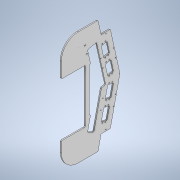
# Autodesk Inventor part: main
Saved by Autodesk Inventor 2020 (Build 240168000, 168)
## iProperties
Created: 2019-06-06
Part Number: main
Material: Generic
Document SubType Name: Modeling
Designer: Vivek Muskan
Density: 1 g/cm^3
Appearance: Default
Author: Vivek Muskan
Autodesk Inventor part; units mm, degrees
ref_plane "XZ Plane" through (0, 0, 0) normal (0, 1, 0) x (-1, 0, 0)
ref_plane "XY Plane" through (0, 0, 0) normal (0, 0, 1) x (1, 0, 0)
sketch "Sketch1" plane through (0, 0, 0) normal (1, 0, 0) x (0, 1, 0)
  line L0 (95.3933, 128.2999) -> (96.692, 122.4421)
  line L1 (96.692, 122.4421) -> (138.1845, 131.641)
  line L2 (138.1845, 131.641) -> (136.8858, 137.4987)
  line L3 (136.8858, 137.4987) -> (139.8147, 138.1481)
  line L4 (139.8147, 138.1481) -> (141.936, 128.5799)
  line L5 (141.936, 128.5799) -> (92.3267, 117.5816)
  line L6 (92.3267, 117.5816) -> (88.0247, 117.5816)
  spline S0 degree 3 poles (88.0247, 117.5816) (88.0217, 119.2517) (88.0187, 120.9217) (88.0127, 124.2551) (88.0097, 125.9183) (88.0067, 127.5816) knots 0.001058 0.001058 0.001058 0.001058 0.502075 0.502075 1.00106 1.00106 1.00106 1.00106
  line L7 (88.0067, 127.5816) -> (92.1535, 127.5816)
  line L8 (92.1535, 127.5816) -> (95.3933, 128.2999)
  line L9 (194.3215, 144.0865) -> (193.0228, 149.9442)
  line L10 (193.0228, 149.9442) -> (196.2626, 150.6625)
  line L11 (196.2626, 150.6625) -> (200.021, 152.4151)
  spline S1 degree 3 poles (200.021, 152.4151) (200.7212, 150.9064) (201.4214, 149.3977) (202.8247, 146.3741) (203.5278, 144.8593) (204.2309, 143.3444) knots 0.003093 0.003093 0.003093 0.003093 0.502078 0.502078 1.003095 1.003095 1.003095 1.003095
  line L12 (204.2309, 143.3444) -> (200.3319, 141.5262)
  line L13 (200.3319, 141.5262) -> (150.7226, 130.5279)
  line L14 (150.7226, 130.5279) -> (148.6014, 140.0961)
  line L15 (148.6014, 140.0961) -> (151.5303, 140.7454)
  line L16 (151.5303, 140.7454) -> (152.8289, 134.8876)
  line L17 (152.8289, 134.8876) -> (194.3215, 144.0865)
  line L18 (-17.9716, 149.9442) -> (-19.2702, 144.0865)
  line L19 (-19.2702, 144.0865) -> (22.2223, 134.8876)
  line L20 (22.2223, 134.8876) -> (23.521, 140.7454)
  line L21 (23.521, 140.7454) -> (26.4499, 140.0961)
  line L22 (26.4499, 140.0961) -> (24.3286, 130.5279)
  line L23 (24.3286, 130.5279) -> (-25.2806, 141.5262)
  line L24 (-25.2806, 141.5262) -> (-21.2113, 150.6625)
  line L25 (-21.2113, 150.6625) -> (-17.9716, 149.9442)
  line L26 (78.3593, 122.4421) -> (79.658, 128.2999)
  line L27 (79.658, 128.2999) -> (82.8977, 127.5816)
  line L28 (82.8977, 127.5816) -> (82.7245, 117.5816)
  line L29 (82.7245, 117.5816) -> (33.1153, 128.5799)
  line L30 (33.1153, 128.5799) -> (35.2365, 138.1481)
  line L31 (35.2365, 138.1481) -> (38.1654, 137.4987)
  line L32 (38.1654, 137.4987) -> (36.8667, 131.641)
  line L33 (36.8667, 131.641) -> (78.3593, 122.4421)
  arc A0 (139.2327, 145.3934) -> (138.4729, 144.2007) centre (139.4492, 144.4171) ccw
  line L34 (139.2327, 145.3934) -> (139.9948, 141.9562)
  ellipse E0 centre (143.732, 141.2695) end of major axis (123.0936, 136.694) minor radius 1.5 (139.9948, 141.9562) -> (139.0214, 141.7264) ccw
  line L35 (139.0214, 141.7264) -> (138.4729, 144.2007)
  arc A1 (147.2595, 146.1487) -> (146.0668, 146.9085) centre (146.2832, 145.9322) ccw
  line L36 (147.2595, 146.1487) -> (147.8081, 143.6744)
  ellipse E1 centre (143.732, 141.2695) end of major axis (123.0936, 136.694) minor radius 1.5 (147.8081, 143.6744) -> (146.8288, 143.4713) ccw
  line L37 (146.8288, 143.4713) -> (146.0668, 146.9085)
  arc A2 (133.4164, 118.4969) -> (134.6092, 117.7371) centre (134.3927, 118.7134) ccw
  line L38 (133.4164, 118.4969) -> (137.0323, 119.2986)
  line L39 (137.0323, 119.2986) -> (137.2487, 118.3223)
  line L40 (137.2487, 118.3223) -> (134.6092, 117.7371)
  arc A3 (161.9454, 123.7975) -> (162.7053, 124.9902) centre (161.729, 124.7738) ccw
  line L41 (161.9454, 123.7975) -> (159.3059, 123.2123)
  line L42 (159.3059, 123.2123) -> (159.0894, 124.1886)
  line L43 (159.0894, 124.1886) -> (162.7053, 124.9902)
  line L44 (156.7254, 122.6402) -> (152.6706, 121.7413)
  arc A4 (151.4779, 122.5011) -> (152.6706, 121.7413) centre (152.4542, 122.7176) ccw
  line L45 (151.4779, 122.5011) -> (147.4692, 140.5828)
  ellipse E2 centre (143.732, 141.2695) end of major axis (123.0936, 136.694) minor radius 1.5 (147.4692, 140.5828) -> (148.4425, 140.8126) ccw
  line L46 (148.4425, 140.8126) -> (152.4542, 122.7176)
  line L47 (152.4542, 122.7176) -> (156.509, 123.6165)
  line L48 (156.509, 123.6165) -> (156.7254, 122.6402)
  line L49 (143.884, 119.7933) -> (139.8292, 118.8943)
  line L50 (139.8292, 118.8943) -> (139.6127, 119.8706)
  line L51 (139.6127, 119.8706) -> (143.6675, 120.7696)
  line L52 (143.6675, 120.7696) -> (139.6559, 138.8646)
  ellipse E3 centre (143.732, 141.2695) end of major axis (123.0936, 136.694) minor radius 1.5 (139.6559, 138.8646) -> (140.6351, 139.0677) ccw
  line L53 (140.6351, 139.0677) -> (144.6438, 120.986)
  arc A5 (143.884, 119.7933) -> (144.6438, 120.986) centre (143.6675, 120.7696) ccw
  ellipse E4 centre (161.9564, 59.0659) end of major axis (159.5624, 58.5351) minor radius 1.5 (164.0969, 58.6514) -> (163.7212, 60.3461) ccw
  line L54 (163.7212, 60.3461) -> (147.4307, 133.8261)
  ellipse E5 centre (145.2903, 134.2406) end of major axis (142.8962, 133.7098) minor radius 1.5 (147.4307, 133.8261) -> (147.055, 135.5208) ccw
  line L55 (147.055, 135.5208) -> (146.1607, 139.5549)
  line L56 (146.1607, 139.5549) -> (147.6251, 139.8796)
  line L57 (147.6251, 139.8796) -> (153.4691, 113.5196)
  line L58 (153.4691, 113.5196) -> (153.9572, 113.6279)
  line L59 (153.9572, 113.6279) -> (165.3205, 62.3724)
  line L60 (165.3205, 62.3724) -> (166.7849, 62.697)
  arc A6 (167.3813, 62.3171) -> (166.7849, 62.697) centre (166.8932, 62.2089) ccw
  line L61 (167.3813, 62.3171) -> (168.2471, 58.4119)
  arc A7 (167.8672, 57.8156) -> (168.2471, 58.4119) centre (167.7589, 58.3037) ccw
  line L62 (167.8672, 57.8156) -> (166.4027, 57.4909)
  line L63 (166.4027, 57.4909) -> (175.6016, 15.9983)
  line L64 (176.6838, 11.1169) -> (175.6016, 15.9983)
  line L65 (168.8734, 9.3853) -> (176.6838, 11.1169)
  line L66 (167.7912, 14.2668) -> (168.8734, 9.3853)
  line L67 (166.3268, 13.9421) -> (167.7912, 14.2668)
  arc A8 (166.3268, 13.9421) -> (165.9468, 13.3458) centre (166.435, 13.454) ccw
  line L68 (166.8126, 9.4406) -> (165.9468, 13.3458)
  arc A9 (166.8126, 9.4406) -> (167.409, 9.0607) centre (167.3008, 9.5488) ccw
  line L69 (168.8734, 9.3853) -> (167.409, 9.0607)
  line L70 (173.649, 15.5655) -> (164.0969, 58.6514)
  line L71 (175.6016, 15.9983) -> (173.649, 15.5655)
  line L72 (175.6016, 15.9983) -> (177.066, 16.323)
  arc A10 (177.6624, 15.9431) -> (177.066, 16.323) centre (177.1742, 15.8349) ccw
  line L73 (177.6624, 15.9431) -> (178.5282, 12.0379)
  arc A11 (178.1482, 11.4415) -> (178.5282, 12.0379) centre (178.04, 11.9297) ccw
  line L74 (178.1482, 11.4415) -> (176.6838, 11.1169)
  line L75 (176.6838, 11.1169) -> (177.0489, 9.4698)
  spline S2 degree 3 poles (177.0489, 9.4698) (177.3581, 9.4352) (177.6662, 9.3893) (177.9705, 9.3319) knots 0 0 0 0 1 1 1 1
  spline S3 degree 3 poles (177.9705, 9.3319) (178.4794, 9.1196) (178.9465, 8.8214) (179.6554, 8.1062) (179.9121, 7.7265) (180.2441, 6.9075) (180.3244, 6.4875) (180.3196, 5.6166) (180.2281, 5.1807) (179.874, 4.3056) (179.5974, 3.8854) (179.26, 3.5154) knots 0 0 0 0 0.165421 0.165421 0.303246 0.303246 0.432052 0.432052 0.565959 0.565959 0.716299 0.716299 0.716299 0.716299
  spline S4 degree 3 poles (179.26, 3.5154) (179.0084, 3.3348) (178.7486, 3.163) (178.4831, 3.001) knots 0 0 0 0 1 1 1 1
  line L76 (178.4831, 3.001) -> (178.8482, 1.3539)
  line L77 (178.8482, 1.3539) -> (186.6586, 3.0855)
  arc A12 (186.875, 2.1092) -> (186.6586, 3.0855) centre (186.7668, 2.5973) ccw
  line L78 (186.875, 2.1092) -> (163.4439, -3.0855)
  arc A13 (163.2275, -2.1092) -> (163.4439, -3.0855) centre (163.3357, -2.5973) ccw
  line L79 (163.2275, -2.1092) -> (171.0379, -0.3776)
  line L80 (171.0379, -0.3776) -> (170.6727, 1.2695)
  spline S5 degree 3 poles (170.6727, 1.2695) (170.3636, 1.3041) (170.0555, 1.3499) (169.7511, 1.4073) knots 0 0 0 0 1 1 1 1
  spline S6 degree 3 poles (169.7511, 1.4073) (169.2423, 1.6196) (168.7751, 1.9178) (168.0663, 2.633) (167.8096, 3.0127) (167.4776, 3.8317) (167.3972, 4.2517) (167.402, 5.1226) (167.4935, 5.5584) (167.8476, 6.4335) (168.1243, 6.8538) (168.4616, 7.2238) knots 0 0 0 0 0.165416 0.165416 0.303241 0.303241 0.43205 0.43205 0.565943 0.565943 0.716298 0.716298 0.716298 0.716298
  spline S7 degree 3 poles (168.4616, 7.2238) (168.7132, 7.4044) (168.973, 7.5762) (169.2386, 7.7382) knots 0 0 0 0 1 1 1 1
  line L81 (169.2386, 7.7382) -> (168.8734, 9.3853)
  line L82 (167.7912, 14.2668) -> (158.5924, 55.7593)
  line L83 (158.5924, 55.7593) -> (157.1279, 55.4347)
  arc A14 (156.5315, 55.8146) -> (157.1279, 55.4347) centre (157.0197, 55.9228) ccw
  line L84 (156.5315, 55.8146) -> (155.6658, 59.7198)
  arc A15 (156.0457, 60.3162) -> (155.6658, 59.7198) centre (156.1539, 59.828) ccw
  line L85 (156.0457, 60.3162) -> (157.5101, 60.6408)
  line L86 (157.5101, 60.6408) -> (146.1469, 111.8963)
  line L87 (146.1469, 111.8963) -> (146.635, 112.0045)
  line L88 (146.635, 112.0045) -> (140.791, 138.3645)
  line L89 (140.791, 138.3645) -> (142.2555, 138.6892)
  line L90 (142.2555, 138.6892) -> (143.1498, 134.655)
  ellipse E6 centre (145.2903, 134.2406) end of major axis (142.8962, 133.7098) minor radius 1.5 (143.1498, 134.655) -> (143.5255, 132.9603) ccw
  line L91 (143.5255, 132.9603) -> (159.816, 59.4803)
  ellipse E7 centre (161.9564, 59.0659) end of major axis (159.5624, 58.5351) minor radius 1.5 (159.816, 59.4803) -> (160.1917, 57.7856) ccw
  line L92 (160.1917, 57.7856) -> (169.7438, 14.6997)
  line L93 (169.7438, 14.6997) -> (167.7912, 14.2668)
  arc A16 (17.9233, 55.4347) -> (18.5197, 55.8146) centre (18.0316, 55.9228) ccw
  line L94 (17.9233, 55.4347) -> (16.4589, 55.7593)
  line L95 (16.4589, 55.7593) -> (7.2601, 14.2668)
  line L96 (6.1778, 9.3853) -> (7.2601, 14.2668)
  line L97 (-1.6325, 11.1169) -> (6.1778, 9.3853)
  line L98 (-0.5503, 15.9983) -> (-1.6325, 11.1169)
  line L99 (-2.0147, 16.323) -> (-0.5503, 15.9983)
  arc A17 (-2.0147, 16.323) -> (-2.6111, 15.9431) centre (-2.123, 15.8349) ccw
  line L100 (-3.4769, 12.0379) -> (-2.6111, 15.9431)
  arc A18 (-3.4769, 12.0379) -> (-3.097, 11.4415) centre (-2.9887, 11.9297) ccw
  line L101 (-1.6325, 11.1169) -> (-3.097, 11.4415)
  line L102 (19.3855, 59.7198) -> (18.5197, 55.8146)
  arc A19 (19.3855, 59.7198) -> (19.0056, 60.3162) centre (18.8973, 59.828) ccw
  line L103 (17.5411, 60.6408) -> (19.0056, 60.3162)
  line L104 (28.9044, 111.8963) -> (17.5411, 60.6408)
  line L105 (28.4163, 112.0045) -> (28.9044, 111.8963)
  line L106 (34.2602, 138.3645) -> (28.4163, 112.0045)
  line L107 (32.7958, 138.6892) -> (34.2602, 138.3645)
  line L108 (5.3075, 14.6997) -> (32.7958, 138.6892)
  line L109 (7.2601, 14.2668) -> (5.3075, 14.6997)
  line L110 (7.2601, 14.2668) -> (8.7245, 13.9421)
  arc A20 (9.1044, 13.3458) -> (8.7245, 13.9421) centre (8.6163, 13.454) ccw
  line L111 (9.1044, 13.3458) -> (8.2386, 9.4406)
  arc A21 (7.6423, 9.0607) -> (8.2386, 9.4406) centre (7.7505, 9.5488) ccw
  line L112 (7.6423, 9.0607) -> (6.1778, 9.3853)
  line L113 (6.1778, 9.3853) -> (5.6103, 6.8252)
  spline S8 degree 3 poles (5.6103, 6.8252) (5.7286, 6.5778) (5.821, 6.3184) (6.0016, 5.5644) (6.0226, 5.0618) (5.8699, 4.0751) (5.6978, 3.6018) (5.2656, 2.886) (5.0546, 2.6222) (4.7378, 2.3167) (4.6606, 2.248) (4.581, 2.1825) knots 0.072842 0.072842 0.072842 0.072842 0.155722 0.155722 0.305743 0.305743 0.455837 0.455837 0.557008 0.557008 0.58807 0.58807 0.58807 0.58807
  line L114 (4.581, 2.1825) -> (4.0134, -0.3776)
  line L115 (4.0134, -0.3776) -> (11.8238, -2.1092)
  arc A22 (11.6073, -3.0855) -> (11.8238, -2.1092) centre (11.7155, -2.5973) ccw
  line L116 (11.6073, -3.0855) -> (-11.8238, 2.1092)
  arc A23 (-11.6073, 3.0855) -> (-11.8238, 2.1092) centre (-11.7155, 2.5973) ccw
  line L117 (-11.6073, 3.0855) -> (-3.797, 1.3539)
  line L118 (-3.797, 1.3539) -> (-3.2294, 3.9141)
  spline S9 degree 3 poles (-3.2294, 3.9141) (-3.3477, 4.1615) (-3.4402, 4.421) (-3.6207, 5.175) (-3.6417, 5.6777) (-3.489, 6.6644) (-3.3168, 7.1377) (-2.8846, 7.8534) (-2.6737, 8.1171) (-2.3568, 8.4226) (-2.2797, 8.4913) (-2.2001, 8.5567) knots 0.072841 0.072841 0.072841 0.072841 0.155736 0.155736 0.305765 0.305765 0.455858 0.455858 0.557024 0.557024 0.58807 0.58807 0.58807 0.58807
  line L119 (-2.2001, 8.5567) -> (-1.6325, 11.1169)
  line L120 (-0.5503, 15.9983) -> (8.6485, 57.4909)
  line L121 (8.6485, 57.4909) -> (7.1841, 57.8156)
  arc A24 (6.8042, 58.4119) -> (7.1841, 57.8156) centre (7.2923, 58.3037) ccw
  line L122 (6.8042, 58.4119) -> (7.6699, 62.3171)
  arc A25 (8.2663, 62.697) -> (7.6699, 62.3171) centre (8.1581, 62.2089) ccw
  line L123 (8.2663, 62.697) -> (9.7308, 62.3724)
  line L124 (9.7308, 62.3724) -> (21.094, 113.6279)
  line L125 (21.094, 113.6279) -> (21.5822, 113.5196)
  line L126 (21.5822, 113.5196) -> (27.4262, 139.8796)
  line L127 (27.4262, 139.8796) -> (28.8906, 139.5549)
  line L128 (28.8906, 139.5549) -> (1.4023, 15.5655)
  line L129 (1.4023, 15.5655) -> (-0.5503, 15.9983)
  arc A26 (161.4872, 36.7266) -> (161.6273, 37.6487) centre (161.379, 37.2147) ccw
  line L130 (161.4872, 36.7266) -> (145.1765, 33.1105)
  arc A27 (144.5802, 33.4904) -> (145.1765, 33.1105) centre (145.0683, 33.5987) ccw
  line L131 (144.5802, 33.4904) -> (142.7404, 41.7889)
  arc A28 (143.5002, 42.9817) -> (142.7404, 41.7889) centre (143.7167, 42.0054) ccw
  line L132 (143.5002, 42.9817) -> (149.8462, 44.3886)
  line L133 (149.8462, 44.3886) -> (161.6273, 37.6487)
  arc A29 (171.3062, 39.7945) -> (171.8228, 39.018) centre (171.7146, 39.5061) ccw
  line L134 (171.3062, 39.7945) -> (179.135, 50.8819)
  line L135 (179.135, 50.8819) -> (185.4809, 52.2888)
  arc A30 (186.6737, 51.5289) -> (185.4809, 52.2888) centre (185.6974, 51.3125) ccw
  line L136 (186.6737, 51.5289) -> (188.5134, 43.2304)
  arc A31 (188.1335, 42.634) -> (188.5134, 43.2304) centre (188.0253, 43.1222) ccw
  line L137 (188.1335, 42.634) -> (171.8228, 39.018)
  line L138 (161.0183, 44.8169) -> (164.9858, 26.9211)
  arc A32 (161.0183, 44.8169) -> (164.9858, 26.9211) centre (166.9072, 36.7347) ccw
  line L139 (172.7961, 28.6526) -> (168.8287, 46.5484)
  arc A33 (172.7961, 28.6526) -> (168.8287, 46.5484) centre (166.9072, 36.7347) ccw
  line L140 (150.4699, 30.7267) -> (149.7182, 34.1174)
  line L141 (149.7182, 34.1174) -> (157.0404, 35.7407)
  arc A34 (157.0404, 35.7407) -> (157.7921, 32.3501) centre (167.0309, 36.1769) ccw
  line L142 (157.7921, 32.3501) -> (150.4699, 30.7267)
  line L143 (183.5919, 41.6271) -> (184.3436, 38.2365)
  line L144 (184.3436, 38.2365) -> (177.0214, 36.6132)
  arc A35 (177.0214, 36.6132) -> (176.2697, 40.0038) centre (167.0309, 36.1769) ccw
  line L145 (176.2697, 40.0038) -> (183.5919, 41.6271)
  arc A36 (7.0216, 56.1278) -> (7.5383, 56.9044) centre (7.1299, 56.616) ccw
  line L146 (7.0216, 56.1278) -> (-9.289, 59.7439)
  arc A37 (-9.669, 60.3402) -> (-9.289, 59.7439) centre (-9.1808, 60.232) ccw
  line L147 (-9.669, 60.3402) -> (-7.8292, 68.6387)
  arc A38 (-6.6364, 69.3986) -> (-7.8292, 68.6387) centre (-6.8529, 68.4223) ccw
  line L148 (-6.6364, 69.3986) -> (-0.2905, 67.9917)
  line L149 (-0.2905, 67.9917) -> (7.5383, 56.9044)
  arc A39 (17.2172, 54.7586) -> (17.3573, 53.8364) centre (17.4655, 54.3246) ccw
  line L150 (17.2172, 54.7586) -> (28.9983, 61.4984)
  line L151 (28.9983, 61.4984) -> (35.3442, 60.0915)
  arc A40 (36.1041, 58.8988) -> (35.3442, 60.0915) centre (35.1278, 59.1152) ccw
  line L152 (36.1041, 58.8988) -> (34.2643, 50.6003)
  arc A41 (33.668, 50.2204) -> (34.2643, 50.6003) centre (33.7762, 50.7085) ccw
  line L153 (33.668, 50.2204) -> (17.3573, 53.8364)
  line L154 (13.8587, 44.0309) -> (17.8262, 61.9267)
  arc A42 (13.8587, 44.0309) -> (17.8262, 61.9267) centre (11.9373, 53.8446) ccw
  line L155 (10.0158, 63.6582) -> (6.0484, 45.7625)
  arc A43 (10.0158, 63.6582) -> (6.0484, 45.7625) centre (11.9373, 53.8446) ccw
  line L156 (-5.4991, 55.3464) -> (-4.7474, 58.737)
  line L157 (-4.7474, 58.737) -> (2.5748, 57.1137)
  arc A44 (2.5748, 57.1137) -> (1.8231, 53.723) centre (11.8136, 53.2868) ccw
  line L158 (1.8231, 53.723) -> (-5.4991, 55.3464)
  line L159 (29.1263, 51.2272) -> (28.3746, 47.8366)
  line L160 (28.3746, 47.8366) -> (21.0524, 49.4599)
  arc A45 (21.0524, 49.4599) -> (21.8041, 52.8506) centre (11.8136, 53.2868) ccw
  line L161 (21.8041, 52.8506) -> (29.1263, 51.2272)
  line L162 (236.3162, 161.7953) -> (244.9739, 122.7435)
  line L163 (244.9739, 122.7435) -> (234.03, 120.3172)
  line L164 (234.03, 120.3172) -> (225.3723, 159.369)
  line L165 (225.3723, 159.369) -> (236.3162, 161.7953)
  line L166 (217.8904, 116.7391) -> (209.2326, 155.7909)
  line L167 (209.2326, 155.7909) -> (219.8253, 158.1393)
  line L168 (219.8253, 158.1393) -> (228.4831, 119.0875)
  line L169 (228.4831, 119.0875) -> (217.8904, 116.7391)
  line L170 (84.0256, 102.4256) -> (81.8611, 112.1886)
  line L171 (81.8611, 112.1886) -> (139.6564, 125.0017)
  line L172 (139.6564, 125.0017) -> (140.7386, 120.1203)
  line L173 (140.7386, 120.1203) -> (128.5349, 117.4147)
  line L174 (128.5349, 117.4147) -> (129.6172, 112.5332)
  line L175 (129.6172, 112.5332) -> (84.0256, 102.4256)
  line L176 (212.0962, 141.0615) -> (214.2606, 131.2986)
  line L177 (214.2606, 131.2986) -> (168.669, 121.191)
  line L178 (168.669, 121.191) -> (167.5868, 126.0724)
  line L179 (167.5868, 126.0724) -> (155.3831, 123.3669)
  line L180 (155.3831, 123.3669) -> (154.3008, 128.2484)
  line L181 (154.3008, 128.2484) -> (212.0962, 141.0615)
  point P0 (0, 0)
  point P1 (108.9087, 474.0736)
  constraints: 364 end point, 92 point on circle, 46 centre point, 58 other
ref_plane "Work Plane1" through (0, 0, 0) normal (1, 0, 0) x (0, 1, 0)
sketch "Sketch2" plane through (0, 0, 0) normal (1, 0, 0) x (0, 1, 0)
  line L0 (156.5294, 113.7862) -> (78.4257, 96.471)
  line L1 (156.5294, 113.7862) -> (236.5294, 113.7862) construction
  line L2 (78.4257, 96.471) -> (75.1791, 111.1155)
  line L3 (75.1791, 111.1155) -> (-46.8579, 138.1704)
  line L4 (-46.8579, 138.1704) -> (-36.438, 160.8954)
  line L5 (-36.438, 160.8954) -> (90.4805, 132.7583)
  line L6 (-36.438, 160.8954) -> (93.562, 160.8954) construction
  line L7 (90.4805, 132.7583) -> (217.399, 160.8954)
  line L8 (217.399, 160.8954) -> (224.5021, 128.8554)
  line L9 (156.5294, 113.7862) -> (224.5021, 128.8554)
  line L10 (156.5294, 113.7862) -> (256.6588, 113.7862) construction
  line L11 (217.399, 160.8954) -> (217.399, 170.8954)
  line L12 (168.1506, 63.8448) -> (89.9746, 46.5136)
  line L13 (168.1506, 63.8448) -> (267.4189, 63.8448) construction
  line L14 (89.9746, 46.5136) -> (239.9746, 79.7678)
  line L15 (19.6493, 62.1044) -> (89.9746, 46.5136)
  line L16 (19.6493, 62.1044) -> (109.2809, 62.1044) construction
  circle A0 centre (400.6229, 80.1044) radius 7.5
  line L17 (390.1229, 116.1044) -> (390.1229, 65.1044)
  line L18 (390.1229, 65.1044) -> (393.8934, 65.1044)
  arc A1 (396.3525, 65.1044) -> (393.8934, 65.1044) centre (395.1229, 66.6818) ccw
  line L19 (396.3525, 65.1044) -> (403.8934, 65.1044)
  arc A2 (406.3525, 65.1044) -> (403.8934, 65.1044) centre (405.1229, 66.6818) ccw
  line L20 (406.3525, 65.1044) -> (411.1229, 65.1044)
  line L21 (411.1229, 65.1044) -> (411.1229, 116.1044)
  line L22 (411.1229, 116.1044) -> (406.3525, 116.1044)
  arc A3 (403.8934, 116.1044) -> (406.3525, 116.1044) centre (405.1229, 114.527) ccw
  line L23 (403.8934, 116.1044) -> (396.3525, 116.1044)
  arc A4 (393.8934, 116.1044) -> (396.3525, 116.1044) centre (395.1229, 114.527) ccw
  line L24 (393.8934, 116.1044) -> (390.1229, 116.1044)
  circle A5 centre (400.6229, 80.1044) radius 2.5
  circle A6 centre (400.6229, 80.1044) radius 4
  circle A7 centre (400.6229, 80.1044) radius 1.5
  line L25 (161.9554, 58.7505) -> (161.1691, 62.297)
  line L26 (161.9554, 58.7505) -> (165.5881, 58.7505) construction
  line L27 (161.1691, 62.297) -> (149.6439, 59.742)
  line L28 (149.6439, 59.742) -> (147.9124, 67.5523)
  line L29 (147.9124, 67.5523) -> (159.4376, 70.1074)
  line L30 (159.4376, 70.1074) -> (161.1691, 62.297)
  line L31 (152.518, 79.1195) -> (145.6839, 77.6044)
  line L32 (145.6839, 77.6044) -> (105.6558, 68.7304)
  line L33 (105.6558, 68.7304) -> (101.1106, 89.2326)
  line L34 (101.1106, 89.2326) -> (141.1387, 98.1066)
  line L35 (141.1387, 98.1066) -> (145.6839, 77.6044)
  line L36 (105.6558, 68.7304) -> (104.5736, 73.6119)
  line L37 (104.5736, 73.6119) -> (100.6684, 72.7461)
  circle A8 centre (100.6684, 72.7461) radius 2
  line L38 (125.6699, 73.1674) -> (121.1246, 93.6696)
  line L39 (143.4113, 87.8555) -> (103.3832, 78.9815)
  circle A9 centre (98.2876, 83.4854) radius 2
  circle A10 centre (148.5069, 83.3516) radius 2
  circle A11 centre (146.1261, 94.0909) radius 2
  line L40 (168.7343, 82.7146) -> (208.7625, 91.5886)
  line L41 (208.7625, 91.5886) -> (204.2172, 112.0908)
  line L42 (204.2172, 112.0908) -> (164.1891, 103.2168)
  line L43 (164.1891, 103.2168) -> (168.7343, 82.7146)
  circle A12 centre (211.5855, 97.3358) radius 2
  circle A13 centre (209.2046, 108.0751) radius 2
  circle A14 centre (161.3661, 97.4695) radius 2
  circle A15 centre (163.747, 86.7303) radius 2
  line L44 (89.9746, 46.5136) -> (89.9746, 206.5136)
  line L45 (89.9746, 46.5136) -> (249.9746, 46.5136) construction
  line L46 (89.9746, 173.6168) -> (-60.0254, 173.6168)
  line L47 (89.9746, 173.6168) -> (239.9746, 173.6168)
  line L48 (239.9746, 173.6168) -> (239.9746, 79.7678)
  line L49 (143.4113, 87.8555) -> (128.7669, 84.6089)
  circle A16 centre (128.7669, 84.6089) radius 20
  line L50 (218.6287, 157.7106) -> (226.3723, 159.4274)
  line L51 (226.3723, 159.4274) -> (222.5005, 158.569)
  line L52 (222.5005, 158.569) -> (218.4688, 176.7548)
  line L53 (220.9532, 165.5481) -> (235.5977, 168.7947)
  line L54 (220.9532, 165.5481) -> (206.3088, 162.3015)
  circle A17 centre (235.5977, 168.7947) radius 1.5
  circle A18 centre (206.3088, 162.3015) radius 1.5
  line L55 (239.9746, 173.6168) -> (239.9746, 143.6168)
  line L56 (239.9746, 143.6168) -> (239.9746, 112.7363) construction
  line L57 (239.9746, 143.6168) -> (239.9746, 173.6168) construction
  line L58 (161.1691, 62.297) -> (136.7617, 56.8861)
  line L59 (16.0066, 62.812) -> (12.0895, 63.6751)
  line L60 (14.048, 63.2436) -> (38.4624, 57.864)
  arc A19 (38.4624, 57.864) -> (136.7617, 56.8861) centre (88.6642, 163.1322) ccw
  line L61 (161.1691, 62.297) -> (209.9839, 73.119)
  line L62 (239.9746, 112.7363) -> (288.7894, 123.5583)
  line L63 (239.9746, 112.7363) -> (289.9746, 112.7363) construction
  line L64 (218.6287, 157.7106) -> (246.6588, 163.9248)
  line L65 (218.6287, 157.7106) -> (247.3394, 157.7106) construction
  line L66 (246.6588, 163.9248) -> (202.7255, 154.185)
  line L67 (202.7255, 154.185) -> (189.7391, 212.7628)
  line L68 (189.7391, 212.7628) -> (233.6724, 222.5025)
  line L69 (233.6724, 222.5025) -> (246.6588, 163.9248)
  line L70 (288.7894, 123.5583) -> (288.7894, 193.5583)
  line L71 (288.7894, 193.5583) -> (257.1006, 193.5583)
  line L72 (257.1006, 193.5583) -> (187.1006, 193.5583)
  line L73 (183.562, 259.3908) -> (-6.438, 259.3908)
  line L74 (-6.438, 259.3908) -> (-6.438, 339.3908)
  line L75 (-6.438, 339.3908) -> (183.562, 339.3908)
  line L76 (183.562, 339.3908) -> (183.562, 259.3908)
  line L77 (-6.438, 259.3908) -> (93.562, 259.3908)
  line L78 (217.399, 160.8954) -> (168.5842, 150.0734)
  line L79 (168.5842, 150.0734) -> (167.502, 154.9549)
  line L80 (167.502, 154.9549) -> (474.7604, 154.9549) construction
  line L81 (10.6785, 150.4499) -> (15.6785, 150.4499) construction
  line L82 (13.5283, 154.9549) -> (12.3934, 150.0698)
  line L83 (167.502, 154.9549) -> (13.5283, 154.9549)
  line L84 (-19.4051, 157.1193) -> (-129.9935, 157.1193)
  line L85 (288.7894, 193.5583) -> (228.7894, 193.5583)
  line L86 (228.7894, 193.5583) -> (228.7894, 264.4387) construction
  line L87 (228.7894, 193.5583) -> (288.7894, 193.5583) construction
  line L88 (239.9746, 112.7363) -> (395.825, 112.7363) construction
  arc A20 (288.7894, 193.5583) -> (228.7894, 253.5583) centre (228.7894, 193.5583) ccw
  line L89 (228.7894, 253.5583) -> (173.7894, 253.5583)
  line L90 (173.7894, 253.5583) -> (173.7894, 168.5583)
  line L91 (173.7894, 168.5583) -> (-16.2106, 168.5583)
  line L92 (-16.2106, 168.5583) -> (68.7894, 168.5583) construction
  line L93 (239.9746, 112.7363) -> (239.9746, 252.5065)
  line L94 (239.9746, 112.7363) -> (379.7448, 112.7363) construction
  line L95 (239.9746, 252.5065) -> (243.9746, 252.5065)
  line L96 (243.9746, 252.5065) -> (243.9746, 232.5065)
  line L97 (243.9746, 232.5065) -> (239.9746, 232.5065)
  line L98 (161.1691, 62.297) -> (160.5198, 65.2259)
  line L99 (160.5198, 65.2259) -> (143.9228, 61.5465)
  circle A21 centre (143.9228, 61.5465) radius 1.5
  circle A22 centre (177.1168, 68.9054) radius 1.5
  line L100 (89.9746, 46.5136) -> (87.4746, 46.5136)
  line L101 (89.9746, 46.5136) -> (92.4746, 46.5136) construction
  line L102 (87.4746, 46.5136) -> (87.4746, 75.5655)
  line L103 (29.2654, 77.6044) -> (69.2935, 68.7304)
  line L104 (69.2935, 68.7304) -> (73.8387, 89.2326)
  line L105 (73.8387, 89.2326) -> (33.8106, 98.1066)
  line L106 (33.8106, 98.1066) -> (29.2654, 77.6044)
  circle A23 centre (74.2809, 72.7461) radius 2
  circle A24 centre (76.6617, 83.4854) radius 2
  circle A25 centre (28.8232, 94.0909) radius 2
  circle A26 centre (26.4424, 83.3516) radius 2
  line L107 (6.2149, 82.7146) -> (-33.8132, 91.5886)
  circle A27 centre (-36.6362, 97.3358) radius 2
  circle A28 centre (-34.2554, 108.0751) radius 2
  line L108 (-33.8132, 91.5886) -> (-29.268, 112.0908)
  line L109 (-29.268, 112.0908) -> (10.7602, 103.2168)
  circle A29 centre (13.5832, 97.4695) radius 2
  line L110 (10.7602, 103.2168) -> (6.2149, 82.7146)
  circle A30 centre (11.2023, 86.7303) radius 2
  line L111 (-60.0254, 79.5652) -> (-45.4747, 79.5652) construction
  line L112 (84.9746, 46.5136) -> (-65.0254, 79.7678)
  line L113 (-65.0254, 173.6168) -> (-65.0254, 79.7678)
  line L114 (-65.0254, 112.7363) -> (-113.8402, 123.5583)
  line L115 (-113.8402, 123.5583) -> (-113.8402, 193.5583)
  line L116 (-113.8402, 193.5583) -> (-82.1513, 193.5583)
  line L117 (-82.1513, 193.5583) -> (-12.1513, 193.5583)
  arc A31 (-53.8402, 253.5583) -> (-113.8402, 193.5583) centre (-53.8402, 193.5583) ccw
  line L118 (-53.8402, 253.5583) -> (-16.2106, 253.5583)
  line L119 (-65.0254, 112.7363) -> (-65.0254, 252.5065)
  line L120 (-65.0254, 252.5065) -> (-69.0254, 252.5065)
  line L121 (-69.0254, 252.5065) -> (-69.0254, 232.5065)
  line L122 (-69.0254, 232.5065) -> (-65.0254, 232.5065)
  line L123 (-16.2106, 168.5583) -> (-16.2106, 253.5583)
  line L124 (-16.2106, 168.5583) -> (68.7894, 168.5583) construction
  circle A32 centre (31.0265, 61.5465) radius 1.5
  circle A33 centre (-2.1676, 68.9054) radius 1.5
  line L125 (161.1691, 62.297) -> (150.0717, 112.3545)
  line L126 (150.0717, 112.3545) -> (150.721, 109.4257)
  line L127 (150.721, 109.4257) -> (167.2463, 113.4147)
  circle A34 centre (167.2463, 113.4147) radius 1.5
  circle A35 centre (134.0581, 106.0571) radius 1.5
  circle A36 centre (7.7029, 113.4147) radius 1.5
  circle A37 centre (40.8912, 106.0571) radius 1.5
  line L128 (235.5977, 168.7947) -> (235.1648, 170.7473) construction
  line L129 (237.0621, 169.1193) -> (236.6293, 171.0719)
  line L130 (233.7004, 170.4226) -> (234.1332, 168.47)
  arc A38 (234.1332, 168.47) -> (237.0621, 169.1193) centre (235.5977, 168.7947) ccw
  arc A39 (236.6293, 171.0719) -> (233.7004, 170.4226) centre (235.1648, 170.7473) ccw
  line L131 (206.3088, 162.3015) -> (205.8759, 164.2541) construction
  line L132 (207.7732, 162.6261) -> (207.3404, 164.5787)
  line L133 (204.4115, 163.9294) -> (204.8444, 161.9768)
  arc A40 (204.8444, 161.9768) -> (207.7732, 162.6261) centre (206.3088, 162.3015) ccw
  arc A41 (207.3404, 164.5787) -> (204.4115, 163.9294) centre (205.8759, 164.2541) ccw
  line L134 (239.9746, 79.7678) -> (239.9746, 95.7678)
  line L135 (239.9746, 95.7678) -> (234.9746, 95.7678)
  circle A42 centre (234.9746, 95.7678) radius 1.5
  circle A43 centre (-60.0254, 95.7678) radius 1.5
  point P0 (0, 0)
  point P1 (390.1229, 70.1044)
  point P2 (236.9357, 169.4726)
  point P3 (236.9357, 168.1167)
  point P4 (2.8935, 152.1758)
  point P5 (198.4176, 173.6168)
  point P6 (239.9746, 162.4429)
  point P7 (243.9746, 251.6049)
  point P8 (173.7894, 173.6168)
  point P9 (1.1598, 253.5583)
  point P10 (-69.0254, 251.6049)
  point P11 (84.7046, 46.5735)
  point P12 (87.4746, 47.0678)
  point P13 (239.9746, 193.5583)
  point P14 (239.9746, 194.0752)
  point P15 (240.0892, 193.5583)
  point P16 (235.3812, 169.771)
  point P17 (206.0924, 163.2778)
  point P18 (207.7732, 162.6261)
  point P19 (234.1332, 168.47)
  dimension "d1" = 80
  dimension "d2" = 167.5
  dimension "d3" = 15
  dimension "d4" = 125
  dimension "d6" = 25
  dimension "d7" = 130
  dimension "d8" = 12.5
  dimension "d9" = 130
  dimension "d10" = 155
  dimension "d11" = 12.5
  dimension "d12" = 10
  dimension "d14" = 167.5
  dimension "d15" = 0
  dimension "d16" = 12.5
  dimension "d20" = 102.5
  dimension "d21" = 8
  dimension "d22" = 7
  dimension "d23" = 41
  dimension "d24" = 21
  dimension "d25" = 5
  dimension "d26" = 4
  dimension "d27" = 90
  dimension "d28" = 4
  dimension "d29" = 160
  dimension "d30" = 90
  dimension "d32" = 150
  dimension "d35" = 15
  dimension "d36" = 40
  dimension "d38" = 15
  dimension "d39" = 15
  dimension "d40" = 3
  dimension "d41" = 3
  dimension "d42" = 30
  dimension "d43" = 180
  dimension "d50" = 25
  dimension "d51" = 25
  dimension "d52" = 50
  dimension "d53" = 50
  dimension "d54" = 12.5
  dimension "d55" = 12.5
  dimension "d56" = 45
  dimension "d57" = 60
  dimension "d58" = 70
  dimension "d61" = 70
  dimension "d65" = 190
  dimension "d68" = 100
  dimension "d69" = 50
  dimension "d70" = 5
  dimension "d75" = 12.5
  dimension "d79" = 60
  dimension "d80" = 90
  dimension "d82" = 55
  dimension "d87" = 85
  dimension "d88" = 190
  dimension "d91" = 90
  dimension "d92" = 4
  dimension "d93" = 20
  dimension "d94" = 90
  dimension "d97" = 3
  dimension "d98" = 17
  dimension "d99" = 3
  dimension "d100" = 2.5
  dimension "d101" = 180
  dimension "d103" = 85
  constraints: 276 end point, 49 symmetric about line, 44 centre point, 25 horizontal, 25 point on circle, 23 point on line, 17 perpendicular, 13 parallel, 10 coincident, 9 equal length, 8 midpoint, 8 tangent, 4 vertical, 23 other
  measures "d1" distance of L0.start L0.end
  measures "d2" angle of L0 L1
  measures "d3" distance of L0.end L2.end
  measures "d4" distance of L2.end L3.end
  measures "d6" distance of L3.end L4.end
  measures "d7" distance of L4.end L5.end
  measures "d8" angle of L5 L6
  measures "d9" distance of L5.end L7.end
  measures "d10" angle of L7 L5
  measures "d11" angle of L10 L9
  measures "d12" distance of L7.end L11.end
  measures "d14" angle of L12 L13
  measures "d15" distance between parallel lines of L14 L12
  measures "d16" angle of L15 L16
  measures "d20" angle of L26 L25
  measures "d21" distance of L27.end L28.end
  measures "d22" distance of L31.start L31.end
  measures "d23" distance of L31.end L32.end
  measures "d24" distance of L32.end L33.end
  measures "d25" distance of L32.end L36.end
  measures "d26" distance of L36.end L37.end
  measures "d27" angle of L37 L36
  measures "d28" diameter of A8
  measures "d29" distance of L12.end L44.end
  measures "d30" angle of L45 L44
  measures "d32" distance of L46.start L47.end
  measures "d35" distance of L39.start L49.end
  measures "d36" diameter of A16
  measures "d38" distance of L53.start L53.end
  measures "d39" distance of L53.start L54.end
  measures "d40" diameter of A17
  measures "d41" diameter of A18
  measures "d42" distance of L47.end L55.end
  measures "d43" angle of L57 L56
  measures "d50" distance of L25.end L58.end
  measures "d51" distance of L60.start L60.end
  measures "d52" distance of L25.end L61.end
  measures "d53" distance of L56.end L62.end
  measures "d54" angle of L63 L62
  measures "d55" angle of L65 L64
  measures "d56" distance of L64.end L66.end
  measures "d57" distance of L66.end L67.end
  measures "d58" distance of L62.end L70.end
  measures "d61" distance of L71.end L72.end
  measures "d65" distance of L74.end L75.end
  measures "d68" distance of L73.end L77.end
  measures "d69" distance of L7.end L78.end
  measures "d70" distance of L78.end L79.end
  measures "d75" angle of L7 L83
  measures "d79" distance of L70.end L85.end
  measures "d80" angle of L87 L86
  measures "d82" distance of L89.start L89.end
  measures "d87" distance of L89.end L90.end
  measures "d88" distance of L90.end L91.end
  measures "d91" angle of L94 L93
  measures "d92" distance of L93.end L95.end
  measures "d93" distance of L95.end L96.end
  measures "d94" angle of L95 L96
  measures "d97" distance of L25.end L98.end
  measures "d98" distance of L98.end L99.end
  measures "d99" diameter of A21
  measures "d100" distance of L12.end L100.end
  measures "d101" angle of L100 L101
  measures "d103" distance of L118.end L91.end
extrude "Extrusion6" add sketch "Sketch2" along normal blind 4 contours L9 L8 L66 L50 L64 L48 L14 L12 L30 L125 L0 | L125 L29 L28 L12 L44 L0 | L44 L15 L102 A19 L112 L113 L84 L4 L3 L2 L0 | L8 L11 L54 L52 L50 L66 | A19 L100 | L30 L99 L28 L29 | L7 L67 L47 L52 L54 L11 | L5 L4 L84 L113 L119 L117 L123 L91 L44 L83 L82 | L44 L91 L90 L47 L67 L7 L79 L83 | L30 L12 L28 L99 | L52 L47 L48 L64 L50 | L67 L72 L93 L47 | L47 L90 L89 A20 L93 L69 L68 L67 | L67 L68 L69 L93 L72 | L64 L69 L72 L71 L70 L62 L48 | L48 L93 L72 L69 L64 | L113 L114 L115 L84 | L84 L115 L116 L117 L119 L113 | L117 L119 A31 L118 L123 | L69 L93 L97 L96 A20 L71 L72 | A31 L121 L122 L119 L117 L116 | A16 L32 L31 | L31 L35 L34 A16 A11 A10 | A17 L130 A39 L129 | A18 L133 A41 L132 | A42 | A43
extrude "Extrusion7" cut sketch "Sketch2" along normal blind 5 contours A17 L130 A39 L129 | A18 L133 A41 L132
fillet "Fillet1" radius 3 20 edges at (2, 168.5842, 150.0734) (2, 167.502, 154.9549) (2, 217.399, 160.8954) (2, 13.5283, 154.9549) (2, 12.3934, 150.0698) (2, -36.438, 160.8954) (2, -46.8579, 138.1704) (2, 75.1791, 111.1155) (2, 78.4257, 96.471) (2, 224.5021, 128.8554) (2, -16.2106, 168.5583) (2, 173.7894, 168.5583) (2, -113.8402, 123.5583) (2, -65.0254, 79.7678) (2, -65.0254, 112.7363) (2, 239.9746, 79.7678) (2, 239.9746, 112.7363) (2, 288.7894, 123.5583) (2, 173.7894, 253.5583) (2, -16.2106, 253.5583)
fillet "Fillet2" radius 1 16 edges at (2, 204.2172, 112.0908) (2, 208.7625, 91.5886) (2, 168.7343, 82.7146) (2, 164.1891, 103.2168) (2, 145.6839, 77.6044) (2, 105.6558, 68.7304) (2, 101.1106, 89.2326) (2, 141.1387, 98.1066) (2, 69.2935, 68.7304) (2, 73.8387, 89.2326) (2, 29.2654, 77.6044) (2, 33.8106, 98.1066) (2, -33.8132, 91.5886) (2, -29.268, 112.0908) (2, 6.2149, 82.7146) (2, 10.7602, 103.2168)
extrude "Extrusion8" add sketch "Sketch2" along normal blind 4 contours A20 L96 L97 L93 | A31 L119 L122 L121
extrude "Extrusion9" cut sketch "Sketch2" along normal blind 5 contours A42 | A43
body "Solid2"
